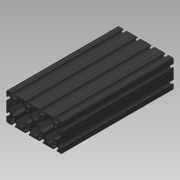
# Autodesk Inventor part: 3060
Saved by Autodesk Inventor 2013 (Build 170138000, 138)
## iProperties
Company: 80/20 Inc.
Created: 2014-04-23
Part Number: 3060
Material: Generic
Document SubType Name: Modeling
Density: 1 g/cm^3
Vendor: 80/20 Inc.
Engineer: Ross Bowman
Designer: Ross Bowman
Catalog Web Link: 8020.net
Material: 6105-T5 Aluminum
Author: Ross Bowman
Keywords: 80/20 , 8020 , T-Slot , Extrusion
Autodesk Inventor part; units mm, degrees
ref_plane "YZ Plane" through (0, 0, 0) normal (1, 0, 0) x (0, 1, 0)
ref_plane "XZ Plane" through (0, 0, 0) normal (0, 1, 0) x (-1, 0, 0)
ref_plane "XY Plane" through (0, 0, 0) normal (0, 0, 1) x (1, 0, 0)
sketch "Sketch1" plane through (0, 0, 0) normal (0, 0, 1) x (1, 0, 0)
  circle A0 centre (57.15, -19.05) radius 3.3274
  circle A1 centre (19.05, -19.05) radius 3.3274
  circle A2 centre (-57.15, 19.05) radius 3.3274
  circle A3 centre (-19.05, 19.05) radius 3.3274
  circle A4 centre (-19.05, -19.05) radius 3.3274
  circle A5 centre (-57.15, -19.05) radius 3.3274
  arc A6 (-51.5823, -18.8539) -> (-50.1854, -22.2287) centre (-46.8071, -18.8539) ccw
  line L0 (-51.5823, -15.4686) -> (-51.5823, -18.8539)
  arc A7 (-51.5823, -15.4686) -> (-54.7573, -12.2936) centre (-54.7573, -15.4686) ccw
  line L1 (-58.1099, -12.2936) -> (-54.7573, -12.2936)
  arc A8 (-61.4883, -10.8932) -> (-58.1099, -12.2936) centre (-58.1099, -7.5184) ccw
  line L2 (-70.3244, -2.0479) -> (-61.4883, -10.8932)
  arc A9 (-70.3244, 2.0479) -> (-70.3244, -2.0479) centre (-68.2744, 0) ccw
  line L3 (-61.4883, 10.8932) -> (-70.3244, 2.0479)
  arc A10 (-58.1099, 12.2936) -> (-61.4883, 10.8932) centre (-58.1099, 7.5184) ccw
  line L4 (-54.7573, 12.2936) -> (-58.1099, 12.2936)
  arc A11 (-54.7573, 12.2936) -> (-51.5823, 15.4686) centre (-54.7573, 15.4686) ccw
  line L5 (-51.5823, 18.8539) -> (-51.5823, 15.4686)
  arc A12 (-50.1854, 22.2287) -> (-51.5823, 18.8539) centre (-46.8071, 18.8539) ccw
  line L6 (-40.8869, 31.5369) -> (-50.1854, 22.2287)
  arc A13 (-36.3704, 31.5369) -> (-40.8869, 31.5369) centre (-38.6286, 29.281) ccw
  line L7 (-27.0718, 22.2287) -> (-36.3704, 31.5369)
  arc A14 (-25.675, 18.8539) -> (-27.0718, 22.2287) centre (-30.4502, 18.8539) ccw
  line L8 (-25.675, 15.4686) -> (-25.675, 18.8539)
  arc A15 (-25.675, 15.4686) -> (-22.5, 12.2936) centre (-22.5, 15.4686) ccw
  line L9 (-19.1368, 12.2936) -> (-22.5, 12.2936)
  arc A16 (-15.7765, 10.9007) -> (-19.1368, 12.2936) centre (-19.1368, 7.5438) ccw
  line L10 (-6.9329, 2.0479) -> (-15.7765, 10.9007)
  arc A17 (-6.9329, -2.0479) -> (-6.9329, 2.0479) centre (-8.9829, 0) ccw
  line L11 (-15.7765, -10.9007) -> (-6.9329, -2.0479)
  arc A18 (-19.1368, -12.2936) -> (-15.7765, -10.9007) centre (-19.1368, -7.5438) ccw
  line L12 (-22.5, -12.2936) -> (-19.1368, -12.2936)
  arc A19 (-22.5, -12.2936) -> (-25.675, -15.4686) centre (-22.5, -15.4686) ccw
  line L13 (-25.675, -18.8539) -> (-25.675, -15.4686)
  arc A20 (-27.0718, -22.2287) -> (-25.675, -18.8539) centre (-30.4502, -18.8539) ccw
  line L14 (-36.3704, -31.5369) -> (-27.0718, -22.2287)
  arc A21 (-40.8869, -31.5369) -> (-36.3704, -31.5369) centre (-38.6286, -29.281) ccw
  line L15 (-50.1854, -22.2287) -> (-40.8869, -31.5369)
  arc A22 (-3.7429, 5.5394) -> (3.7429, 5.5394) centre (0, 9.2784) ccw
  line L16 (-11.3507, 13.1551) -> (-3.7429, 5.5394)
  arc A23 (-12.425, 15.7507) -> (-11.3507, 13.1551) centre (-8.7523, 15.7507) ccw
  line L17 (-12.425, 22.3493) -> (-12.425, 15.7507)
  arc A24 (-11.3507, 24.9449) -> (-12.425, 22.3493) centre (-8.7523, 22.3493) ccw
  line L18 (-2.7156, 33.589) -> (-11.3507, 24.9449)
  arc A25 (2.7156, 33.589) -> (-2.7156, 33.589) centre (0, 30.8762) ccw
  line L19 (11.3507, 24.9449) -> (2.7156, 33.589)
  arc A26 (12.425, 22.3493) -> (11.3507, 24.9449) centre (8.7523, 22.3493) ccw
  line L20 (12.425, 15.7507) -> (12.425, 22.3493)
  arc A27 (11.3507, 13.1551) -> (12.425, 15.7507) centre (8.7523, 15.7507) ccw
  line L21 (3.7429, 5.5394) -> (11.3507, 13.1551)
  circle A28 centre (19.05, 19.05) radius 3.3274
  circle A29 centre (57.15, 19.05) radius 3.3274
  arc A30 (-2.7156, -33.589) -> (2.7156, -33.589) centre (0, -30.8762) ccw
  line L22 (-11.3507, -24.9449) -> (-2.7156, -33.589)
  arc A31 (-12.425, -22.3493) -> (-11.3507, -24.9449) centre (-8.7523, -22.3493) ccw
  line L23 (-12.425, -15.7507) -> (-12.425, -22.3493)
  arc A32 (-11.3507, -13.1551) -> (-12.425, -15.7507) centre (-8.7523, -15.7507) ccw
  line L24 (-3.7429, -5.5394) -> (-11.3507, -13.1551)
  arc A33 (3.7429, -5.5394) -> (-3.7429, -5.5394) centre (0, -9.2784) ccw
  line L25 (11.3507, -13.1551) -> (3.7429, -5.5394)
  arc A34 (12.425, -15.7507) -> (11.3507, -13.1551) centre (8.7523, -15.7507) ccw
  line L26 (12.425, -22.3493) -> (12.425, -15.7507)
  arc A35 (11.3507, -24.9449) -> (12.425, -22.3493) centre (8.7523, -22.3493) ccw
  line L27 (2.7156, -33.589) -> (11.3507, -24.9449)
  arc A36 (6.9329, 2.0479) -> (6.9329, -2.0479) centre (8.9829, 0) ccw
  line L28 (15.7765, 10.9007) -> (6.9329, 2.0479)
  arc A37 (19.1368, 12.2936) -> (15.7765, 10.9007) centre (19.1368, 7.5438) ccw
  line L29 (22.5, 12.2936) -> (19.1368, 12.2936)
  arc A38 (22.5, 12.2936) -> (25.675, 15.4686) centre (22.5, 15.4686) ccw
  line L30 (25.675, 18.8539) -> (25.675, 15.4686)
  arc A39 (27.0718, 22.2287) -> (25.675, 18.8539) centre (30.4502, 18.8539) ccw
  line L31 (36.3704, 31.5369) -> (27.0718, 22.2287)
  arc A40 (40.8869, 31.5369) -> (36.3704, 31.5369) centre (38.6286, 29.281) ccw
  line L32 (50.1854, 22.2287) -> (40.8869, 31.5369)
  arc A41 (51.5823, 18.8539) -> (50.1854, 22.2287) centre (46.8071, 18.8539) ccw
  line L33 (51.5823, 15.4686) -> (51.5823, 18.8539)
  arc A42 (51.5823, 15.4686) -> (54.7573, 12.2936) centre (54.7573, 15.4686) ccw
  line L34 (58.1099, 12.2936) -> (54.7573, 12.2936)
  arc A43 (61.4883, 10.8932) -> (58.1099, 12.2936) centre (58.1099, 7.5184) ccw
  line L35 (70.3244, 2.0479) -> (61.4883, 10.8932)
  arc A44 (70.3244, -2.0479) -> (70.3244, 2.0479) centre (68.2744, 0) ccw
  line L36 (61.4883, -10.8932) -> (70.3244, -2.0479)
  arc A45 (58.1099, -12.2936) -> (61.4883, -10.8932) centre (58.1099, -7.5184) ccw
  line L37 (54.7573, -12.2936) -> (58.1099, -12.2936)
  arc A46 (54.7573, -12.2936) -> (51.5823, -15.4686) centre (54.7573, -15.4686) ccw
  line L38 (51.5823, -18.8539) -> (51.5823, -15.4686)
  arc A47 (50.1854, -22.2287) -> (51.5823, -18.8539) centre (46.8071, -18.8539) ccw
  line L39 (40.8869, -31.5369) -> (50.1854, -22.2287)
  arc A48 (36.3704, -31.5369) -> (40.8869, -31.5369) centre (38.6286, -29.281) ccw
  line L40 (27.0718, -22.2287) -> (36.3704, -31.5369)
  arc A49 (25.675, -18.8539) -> (27.0718, -22.2287) centre (30.4502, -18.8539) ccw
  line L41 (25.675, -15.4686) -> (25.675, -18.8539)
  arc A50 (25.675, -15.4686) -> (22.5, -12.2936) centre (22.5, -15.4686) ccw
  line L42 (19.1368, -12.2936) -> (22.5, -12.2936)
  arc A51 (15.7765, -10.9007) -> (19.1368, -12.2936) centre (19.1368, -7.5438) ccw
  line L43 (6.9329, -2.0479) -> (15.7765, -10.9007)
  arc A52 (28.5292, -38.1) -> (27.0066, -38.1) centre (27.7679, -38.1) ccw
  line L44 (28.5292, -38.1) -> (33.4119, -38.1)
  arc A53 (34.9345, -38.1) -> (33.4119, -38.1) centre (34.1732, -38.1) ccw
  line L45 (34.9345, -38.1) -> (42.3228, -38.1)
  arc A54 (43.8453, -38.1) -> (42.3228, -38.1) centre (43.0841, -38.1) ccw
  line L46 (43.8453, -38.1) -> (47.5811, -38.1)
  arc A55 (49.1036, -38.1) -> (47.5811, -38.1) centre (48.3424, -38.1) ccw
  line L47 (49.1036, -38.1) -> (51.5112, -38.1)
  arc A56 (51.5112, -38.1) -> (53.086, -36.5252) centre (51.5112, -36.5252) ccw
  line L48 (53.086, -36.5252) -> (53.086, -35.6108)
  arc A57 (53.086, -35.6108) -> (51.5112, -34.036) centre (51.5112, -35.6108) ccw
  line L49 (51.5112, -34.036) -> (47.752, -34.036)
  arc A58 (46.863, -33.147) -> (47.752, -34.036) centre (47.752, -33.147) ccw
  line L50 (46.863, -33.147) -> (46.863, -32.5952)
  arc A59 (47.1231, -31.967) -> (46.863, -32.5952) centre (47.752, -32.5952) ccw
  line L51 (47.1231, -31.967) -> (51.9086, -27.1764)
  arc A60 (55.2137, -25.8064) -> (51.9086, -27.1764) centre (55.2137, -30.4782) ccw
  line L52 (55.2137, -25.8064) -> (59.0863, -25.8064)
  arc A61 (62.3914, -27.1764) -> (59.0863, -25.8064) centre (59.0863, -30.4782) ccw
  line L53 (62.3914, -27.1764) -> (67.1769, -31.967)
  arc A62 (67.437, -32.5952) -> (67.1769, -31.967) centre (66.548, -32.5952) ccw
  line L54 (67.437, -32.5952) -> (67.437, -33.147)
  arc A63 (66.548, -34.036) -> (67.437, -33.147) centre (66.548, -33.147) ccw
  line L55 (66.548, -34.036) -> (62.7888, -34.036)
  arc A64 (62.7888, -34.036) -> (61.214, -35.6108) centre (62.7888, -35.6108) ccw
  line L56 (61.214, -35.6108) -> (61.214, -36.5252)
  arc A65 (61.214, -36.5252) -> (62.7888, -38.1) centre (62.7888, -36.5252) ccw
  line L57 (62.7888, -38.1) -> (65.1067, -38.1)
  arc A66 (66.6292, -38.1) -> (65.1067, -38.1) centre (65.8679, -38.1) ccw
  line L58 (66.6292, -38.1) -> (71.4582, -38.1)
  arc A67 (72.9807, -38.1) -> (71.4582, -38.1) centre (72.2194, -38.1) ccw
  arc A68 (72.9807, -38.1) -> (76.2, -35.4576) centre (73.0698, -34.9262) ccw
  arc A69 (76.2, -33.935) -> (76.2, -35.4576) centre (76.2, -34.6963) ccw
  line L59 (76.2, -33.935) -> (76.2, -29.2617)
  arc A70 (76.2, -27.7391) -> (76.2, -29.2617) centre (76.2, -28.5004) ccw
  line L60 (76.2, -27.7391) -> (76.2, -24.6888)
  arc A71 (76.2, -24.6888) -> (74.6252, -23.114) centre (74.6252, -24.6888) ccw
  line L61 (74.6252, -23.114) -> (73.7108, -23.114)
  arc A72 (73.7108, -23.114) -> (72.136, -24.6888) centre (73.7108, -24.6888) ccw
  line L62 (72.136, -24.6888) -> (72.136, -29.1294)
  arc A73 (71.3385, -29.9269) -> (72.136, -29.1294) centre (71.3385, -29.1294) ccw
  line L63 (71.3385, -29.9269) -> (71.2424, -29.9269)
  arc A74 (70.6234, -29.6666) -> (71.2424, -29.9269) centre (71.2424, -29.0607) ccw
  line L64 (70.6234, -29.6666) -> (64.1071, -23.1436)
  arc A75 (62.7177, -19.7867) -> (64.1071, -23.1436) centre (67.4675, -19.7867) ccw
  line L65 (62.7177, -19.7867) -> (62.7177, -18.3133)
  arc A76 (64.1071, -14.9564) -> (62.7177, -18.3133) centre (67.4675, -18.3133) ccw
  line L66 (64.1071, -14.9564) -> (70.6297, -8.4271)
  arc A77 (71.2424, -8.1731) -> (70.6297, -8.4271) centre (71.2424, -9.0392) ccw
  line L67 (71.2424, -8.1731) -> (71.3385, -8.1731)
  arc A78 (72.136, -8.9706) -> (71.3385, -8.1731) centre (71.3385, -8.9706) ccw
  line L68 (72.136, -8.9706) -> (72.136, -13.4112)
  arc A79 (72.136, -13.4112) -> (73.7108, -14.986) centre (73.7108, -13.4112) ccw
  line L69 (73.7108, -14.986) -> (74.6252, -14.986)
  arc A80 (74.6252, -14.986) -> (76.2, -13.4112) centre (74.6252, -13.4112) ccw
  line L70 (76.2, -13.4112) -> (76.2, -11.7903)
  arc A81 (76.2, -10.2663) -> (76.2, -11.7903) centre (76.2, -11.0283) ccw
  line L71 (76.2, -10.2663) -> (76.2, -5.4385)
  arc A82 (76.2, -3.9149) -> (76.2, -5.4385) centre (76.2, -4.6767) ccw
  line L72 (76.2, -3.9149) -> (76.2, 3.9149)
  arc A83 (76.2, 5.4385) -> (76.2, 3.9149) centre (76.2, 4.6767) ccw
  line L73 (76.2, 5.4385) -> (76.2, 10.2663)
  arc A84 (76.2, 11.7903) -> (76.2, 10.2663) centre (76.2, 11.0283) ccw
  line L74 (76.2, 11.7903) -> (76.2, 13.4112)
  arc A85 (76.2, 13.4112) -> (74.6252, 14.986) centre (74.6252, 13.4112) ccw
  line L75 (74.6252, 14.986) -> (73.7108, 14.986)
  arc A86 (73.7108, 14.986) -> (72.136, 13.4112) centre (73.7108, 13.4112) ccw
  line L76 (72.136, 13.4112) -> (72.136, 8.9706)
  arc A87 (71.3385, 8.1731) -> (72.136, 8.9706) centre (71.3385, 8.9706) ccw
  line L77 (71.3385, 8.1731) -> (71.2424, 8.1731)
  arc A88 (70.6297, 8.4271) -> (71.2424, 8.1731) centre (71.2424, 9.0392) ccw
  line L78 (70.6297, 8.4271) -> (64.1071, 14.9564)
  arc A89 (62.7177, 18.3133) -> (64.1071, 14.9564) centre (67.4675, 18.3133) ccw
  line L79 (62.7177, 18.3133) -> (62.7177, 19.7867)
  arc A90 (64.1071, 23.1436) -> (62.7177, 19.7867) centre (67.4675, 19.7867) ccw
  line L80 (64.1071, 23.1436) -> (70.6234, 29.6666)
  arc A91 (71.2424, 29.9269) -> (70.6234, 29.6666) centre (71.2424, 29.0607) ccw
  line L81 (71.2424, 29.9269) -> (71.3385, 29.9269)
  arc A92 (72.136, 29.1294) -> (71.3385, 29.9269) centre (71.3385, 29.1294) ccw
  line L82 (72.136, 29.1294) -> (72.136, 24.6888)
  arc A93 (72.136, 24.6888) -> (73.7108, 23.114) centre (73.7108, 24.6888) ccw
  line L83 (73.7108, 23.114) -> (74.6252, 23.114)
  arc A94 (74.6252, 23.114) -> (76.2, 24.6888) centre (74.6252, 24.6888) ccw
  line L84 (76.2, 24.6888) -> (76.2, 27.7391)
  arc A95 (76.2, 29.2617) -> (76.2, 27.7391) centre (76.2, 28.5004) ccw
  line L85 (76.2, 29.2617) -> (76.2, 33.935)
  arc A96 (76.2, 35.4576) -> (76.2, 33.935) centre (76.2, 34.6963) ccw
  arc A97 (76.2, 35.4576) -> (72.9807, 38.1) centre (73.0698, 34.9262) ccw
  arc A98 (71.4582, 38.1) -> (72.9807, 38.1) centre (72.2194, 38.1) ccw
  line L86 (71.4582, 38.1) -> (66.6292, 38.1)
  arc A99 (65.1067, 38.1) -> (66.6292, 38.1) centre (65.8679, 38.1) ccw
  line L87 (65.1067, 38.1) -> (62.7888, 38.1)
  arc A100 (62.7888, 38.1) -> (61.214, 36.5252) centre (62.7888, 36.5252) ccw
  line L88 (61.214, 36.5252) -> (61.214, 35.6108)
  arc A101 (61.214, 35.6108) -> (62.7888, 34.036) centre (62.7888, 35.6108) ccw
  line L89 (62.7888, 34.036) -> (66.548, 34.036)
  arc A102 (67.437, 33.147) -> (66.548, 34.036) centre (66.548, 33.147) ccw
  line L90 (67.437, 33.147) -> (67.437, 32.5952)
  arc A103 (67.1769, 31.967) -> (67.437, 32.5952) centre (66.548, 32.5952) ccw
  line L91 (67.1769, 31.967) -> (62.3914, 27.1764)
  arc A104 (59.0863, 25.8064) -> (62.3914, 27.1764) centre (59.0863, 30.4782) ccw
  line L92 (59.0863, 25.8064) -> (55.2137, 25.8064)
  arc A105 (51.9086, 27.1764) -> (55.2137, 25.8064) centre (55.2137, 30.4782) ccw
  line L93 (51.9086, 27.1764) -> (47.1231, 31.967)
  arc A106 (46.863, 32.5952) -> (47.1231, 31.967) centre (47.752, 32.5952) ccw
  line L94 (46.863, 32.5952) -> (46.863, 33.147)
  arc A107 (47.752, 34.036) -> (46.863, 33.147) centre (47.752, 33.147) ccw
  line L95 (47.752, 34.036) -> (51.5112, 34.036)
  arc A108 (51.5112, 34.036) -> (53.086, 35.6108) centre (51.5112, 35.6108) ccw
  line L96 (53.086, 35.6108) -> (53.086, 36.5252)
  arc A109 (53.086, 36.5252) -> (51.5112, 38.1) centre (51.5112, 36.5252) ccw
  line L97 (51.5112, 38.1) -> (49.1036, 38.1)
  arc A110 (47.5811, 38.1) -> (49.1036, 38.1) centre (48.3424, 38.1) ccw
  line L98 (47.5811, 38.1) -> (43.8453, 38.1)
  arc A111 (42.3228, 38.1) -> (43.8453, 38.1) centre (43.0841, 38.1) ccw
  line L99 (42.3228, 38.1) -> (34.9345, 38.1)
  arc A112 (33.4119, 38.1) -> (34.9345, 38.1) centre (34.1732, 38.1) ccw
  line L100 (33.4119, 38.1) -> (28.5292, 38.1)
  arc A113 (27.0066, 38.1) -> (28.5292, 38.1) centre (27.7679, 38.1) ccw
  line L101 (27.0066, 38.1) -> (24.6888, 38.1)
  arc A114 (24.6888, 38.1) -> (23.114, 36.5252) centre (24.6888, 36.5252) ccw
  line L102 (23.114, 36.5252) -> (23.114, 35.6108)
  arc A115 (23.114, 35.6108) -> (24.6888, 34.036) centre (24.6888, 35.6108) ccw
  line L103 (24.6888, 34.036) -> (28.448, 34.036)
  arc A116 (29.337, 33.147) -> (28.448, 34.036) centre (28.448, 33.147) ccw
  line L104 (29.337, 33.147) -> (29.337, 32.9805)
  arc A117 (29.0769, 32.3522) -> (29.337, 32.9805) centre (28.448, 32.9805) ccw
  line L105 (29.0769, 32.3522) -> (23.9294, 27.1993)
  arc A118 (20.5691, 25.8064) -> (23.9294, 27.1993) centre (20.5691, 30.5562) ccw
  line L106 (20.5691, 25.8064) -> (17.5309, 25.8064)
  arc A119 (14.1706, 27.1993) -> (17.5309, 25.8064) centre (17.5309, 30.5562) ccw
  line L107 (14.1706, 27.1993) -> (9.0231, 32.3522)
  arc A120 (8.763, 32.9805) -> (9.0231, 32.3522) centre (9.652, 32.9805) ccw
  line L108 (8.763, 32.9805) -> (8.763, 33.147)
  arc A121 (9.652, 34.036) -> (8.763, 33.147) centre (9.652, 33.147) ccw
  line L109 (9.652, 34.036) -> (13.4112, 34.036)
  arc A122 (13.4112, 34.036) -> (14.986, 35.6108) centre (13.4112, 35.6108) ccw
  line L110 (14.986, 35.6108) -> (14.986, 36.4702)
  arc A123 (14.986, 36.4702) -> (13.4122, 38.1) centre (13.4122, 36.5252) ccw
  line L111 (13.4122, 38.1) -> (11.0569, 38.1)
  arc A124 (9.5343, 38.1) -> (11.0569, 38.1) centre (10.2956, 38.1) ccw
  line L112 (9.5343, 38.1) -> (4.6578, 38.1)
  arc A125 (3.1353, 38.1) -> (4.6578, 38.1) centre (3.8965, 38.1) ccw
  line L113 (3.1353, 38.1) -> (-3.1353, 38.1)
  arc A126 (-4.6578, 38.1) -> (-3.1353, 38.1) centre (-3.8965, 38.1) ccw
  line L114 (-4.6578, 38.1) -> (-9.5343, 38.1)
  arc A127 (-11.0569, 38.1) -> (-9.5343, 38.1) centre (-10.2956, 38.1) ccw
  line L115 (-11.0569, 38.1) -> (-13.4122, 38.1)
  arc A128 (-13.4122, 38.1) -> (-14.986, 36.4702) centre (-13.4122, 36.5252) ccw
  line L116 (-14.986, 36.4702) -> (-14.986, 35.6108)
  arc A129 (-14.986, 35.6108) -> (-13.4112, 34.036) centre (-13.4112, 35.6108) ccw
  line L117 (-13.4112, 34.036) -> (-9.652, 34.036)
  arc A130 (-8.763, 33.147) -> (-9.652, 34.036) centre (-9.652, 33.147) ccw
  line L118 (-8.763, 33.147) -> (-8.763, 32.9805)
  arc A131 (-9.0231, 32.3522) -> (-8.763, 32.9805) centre (-9.652, 32.9805) ccw
  line L119 (-9.0231, 32.3522) -> (-14.1706, 27.1993)
  arc A132 (-17.5309, 25.8064) -> (-14.1706, 27.1993) centre (-17.5309, 30.5562) ccw
  line L120 (-17.5309, 25.8064) -> (-20.5691, 25.8064)
  arc A133 (-23.9294, 27.1993) -> (-20.5691, 25.8064) centre (-20.5691, 30.5562) ccw
  line L121 (-23.9294, 27.1993) -> (-29.0769, 32.3522)
  arc A134 (-29.337, 32.9805) -> (-29.0769, 32.3522) centre (-28.448, 32.9805) ccw
  line L122 (-29.337, 32.9805) -> (-29.337, 33.147)
  arc A135 (-28.448, 34.036) -> (-29.337, 33.147) centre (-28.448, 33.147) ccw
  line L123 (-28.448, 34.036) -> (-24.6888, 34.036)
  arc A136 (-24.6888, 34.036) -> (-23.114, 35.6108) centre (-24.6888, 35.6108) ccw
  line L124 (-23.114, 35.6108) -> (-23.114, 36.5252)
  arc A137 (-23.114, 36.5252) -> (-24.6888, 38.1) centre (-24.6888, 36.5252) ccw
  line L125 (-24.6888, 38.1) -> (-27.0066, 38.1)
  arc A138 (-28.5292, 38.1) -> (-27.0066, 38.1) centre (-27.7679, 38.1) ccw
  line L126 (-28.5292, 38.1) -> (-33.4119, 38.1)
  arc A139 (-34.9345, 38.1) -> (-33.4119, 38.1) centre (-34.1732, 38.1) ccw
  line L127 (-34.9345, 38.1) -> (-42.3228, 38.1)
  arc A140 (-43.8453, 38.1) -> (-42.3228, 38.1) centre (-43.0841, 38.1) ccw
  line L128 (-43.8453, 38.1) -> (-47.5811, 38.1)
  arc A141 (-49.1036, 38.1) -> (-47.5811, 38.1) centre (-48.3424, 38.1) ccw
  line L129 (-49.1036, 38.1) -> (-51.5112, 38.1)
  arc A142 (-51.5112, 38.1) -> (-53.086, 36.5252) centre (-51.5112, 36.5252) ccw
  line L130 (-53.086, 36.5252) -> (-53.086, 35.6108)
  arc A143 (-53.086, 35.6108) -> (-51.5112, 34.036) centre (-51.5112, 35.6108) ccw
  line L131 (-51.5112, 34.036) -> (-47.752, 34.036)
  arc A144 (-46.863, 33.147) -> (-47.752, 34.036) centre (-47.752, 33.147) ccw
  line L132 (-46.863, 33.147) -> (-46.863, 32.5952)
  arc A145 (-47.1231, 31.967) -> (-46.863, 32.5952) centre (-47.752, 32.5952) ccw
  line L133 (-47.1231, 31.967) -> (-51.9086, 27.1764)
  arc A146 (-55.2137, 25.8064) -> (-51.9086, 27.1764) centre (-55.2137, 30.4782) ccw
  line L134 (-55.2137, 25.8064) -> (-59.0863, 25.8064)
  arc A147 (-62.3914, 27.1764) -> (-59.0863, 25.8064) centre (-59.0863, 30.4782) ccw
  line L135 (-62.3914, 27.1764) -> (-67.1769, 31.967)
  arc A148 (-67.437, 32.5952) -> (-67.1769, 31.967) centre (-66.548, 32.5952) ccw
  line L136 (-67.437, 32.5952) -> (-67.437, 33.147)
  arc A149 (-66.548, 34.036) -> (-67.437, 33.147) centre (-66.548, 33.147) ccw
  line L137 (-66.548, 34.036) -> (-62.7888, 34.036)
  arc A150 (-62.7888, 34.036) -> (-61.214, 35.6108) centre (-62.7888, 35.6108) ccw
  line L138 (-61.214, 35.6108) -> (-61.214, 36.5252)
  arc A151 (-61.214, 36.5252) -> (-62.7888, 38.1) centre (-62.7888, 36.5252) ccw
  line L139 (-62.7888, 38.1) -> (-65.1067, 38.1)
  arc A152 (-66.6292, 38.1) -> (-65.1067, 38.1) centre (-65.8679, 38.1) ccw
  line L140 (-66.6292, 38.1) -> (-71.4582, 38.1)
  arc A153 (-72.9807, 38.1) -> (-71.4582, 38.1) centre (-72.2194, 38.1) ccw
  arc A154 (-72.9807, 38.1) -> (-76.2, 35.4576) centre (-73.0698, 34.9262) ccw
  arc A155 (-76.2, 33.935) -> (-76.2, 35.4576) centre (-76.2, 34.6963) ccw
  line L141 (-76.2, 33.935) -> (-76.2, 29.2617)
  arc A156 (-76.2, 27.7391) -> (-76.2, 29.2617) centre (-76.2, 28.5004) ccw
  line L142 (-76.2, 27.7391) -> (-76.2, 24.6888)
  arc A157 (-76.2, 24.6888) -> (-74.6252, 23.114) centre (-74.6252, 24.6888) ccw
  line L143 (-74.6252, 23.114) -> (-73.7108, 23.114)
  arc A158 (-73.7108, 23.114) -> (-72.136, 24.6888) centre (-73.7108, 24.6888) ccw
  line L144 (-72.136, 24.6888) -> (-72.136, 29.1294)
  arc A159 (-71.3385, 29.9269) -> (-72.136, 29.1294) centre (-71.3385, 29.1294) ccw
  line L145 (-71.3385, 29.9269) -> (-71.2424, 29.9269)
  arc A160 (-70.6234, 29.6666) -> (-71.2424, 29.9269) centre (-71.2424, 29.0607) ccw
  line L146 (-70.6234, 29.6666) -> (-64.1071, 23.1436)
  arc A161 (-62.7177, 19.7867) -> (-64.1071, 23.1436) centre (-67.4675, 19.7867) ccw
  line L147 (-62.7177, 19.7867) -> (-62.7177, 18.3133)
  arc A162 (-64.1071, 14.9564) -> (-62.7177, 18.3133) centre (-67.4675, 18.3133) ccw
  line L148 (-64.1071, 14.9564) -> (-70.6297, 8.4271)
  arc A163 (-71.2424, 8.1731) -> (-70.6297, 8.4271) centre (-71.2424, 9.0392) ccw
  line L149 (-71.2424, 8.1731) -> (-71.3385, 8.1731)
  arc A164 (-72.136, 8.9706) -> (-71.3385, 8.1731) centre (-71.3385, 8.9706) ccw
  line L150 (-72.136, 8.9706) -> (-72.136, 13.4112)
  arc A165 (-72.136, 13.4112) -> (-73.7108, 14.986) centre (-73.7108, 13.4112) ccw
  line L151 (-73.7108, 14.986) -> (-74.6252, 14.986)
  arc A166 (-74.6252, 14.986) -> (-76.2, 13.4112) centre (-74.6252, 13.4112) ccw
  line L152 (-76.2, 13.4112) -> (-76.2, 11.7903)
  arc A167 (-76.2, 10.2663) -> (-76.2, 11.7903) centre (-76.2, 11.0283) ccw
  line L153 (-76.2, 10.2663) -> (-76.2, 5.4385)
  arc A168 (-76.2, 3.9149) -> (-76.2, 5.4385) centre (-76.2, 4.6767) ccw
  line L154 (-76.2, 3.9149) -> (-76.2, -3.9149)
  arc A169 (-76.2, -5.4385) -> (-76.2, -3.9149) centre (-76.2, -4.6767) ccw
  line L155 (-76.2, -5.4385) -> (-76.2, -10.2663)
  arc A170 (-76.2, -11.7903) -> (-76.2, -10.2663) centre (-76.2, -11.0283) ccw
  line L156 (-76.2, -11.7903) -> (-76.2, -13.4112)
  arc A171 (-76.2, -13.4112) -> (-74.6252, -14.986) centre (-74.6252, -13.4112) ccw
  line L157 (-74.6252, -14.986) -> (-73.7108, -14.986)
  arc A172 (-73.7108, -14.986) -> (-72.136, -13.4112) centre (-73.7108, -13.4112) ccw
  line L158 (-72.136, -13.4112) -> (-72.136, -8.9706)
  arc A173 (-71.3385, -8.1731) -> (-72.136, -8.9706) centre (-71.3385, -8.9706) ccw
  line L159 (-71.3385, -8.1731) -> (-71.2424, -8.1731)
  arc A174 (-70.6297, -8.4271) -> (-71.2424, -8.1731) centre (-71.2424, -9.0392) ccw
  line L160 (-70.6297, -8.4271) -> (-64.1071, -14.9564)
  arc A175 (-62.7177, -18.3133) -> (-64.1071, -14.9564) centre (-67.4675, -18.3133) ccw
  line L161 (-62.7177, -18.3133) -> (-62.7177, -19.7867)
  arc A176 (-64.1071, -23.1436) -> (-62.7177, -19.7867) centre (-67.4675, -19.7867) ccw
  line L162 (-64.1071, -23.1436) -> (-70.6234, -29.6666)
  arc A177 (-71.2424, -29.9269) -> (-70.6234, -29.6666) centre (-71.2424, -29.0607) ccw
  line L163 (-71.2424, -29.9269) -> (-71.3385, -29.9269)
  arc A178 (-72.136, -29.1294) -> (-71.3385, -29.9269) centre (-71.3385, -29.1294) ccw
  line L164 (-72.136, -29.1294) -> (-72.136, -24.6888)
  arc A179 (-72.136, -24.6888) -> (-73.7108, -23.114) centre (-73.7108, -24.6888) ccw
  line L165 (-73.7108, -23.114) -> (-74.6252, -23.114)
  arc A180 (-74.6252, -23.114) -> (-76.2, -24.6888) centre (-74.6252, -24.6888) ccw
  line L166 (-76.2, -24.6888) -> (-76.2, -27.7391)
  arc A181 (-76.2, -29.2617) -> (-76.2, -27.7391) centre (-76.2, -28.5004) ccw
  line L167 (-76.2, -29.2617) -> (-76.2, -33.935)
  arc A182 (-76.2, -35.4576) -> (-76.2, -33.935) centre (-76.2, -34.6963) ccw
  arc A183 (-76.2, -35.4576) -> (-72.9807, -38.1) centre (-73.0698, -34.9262) ccw
  arc A184 (-71.4582, -38.1) -> (-72.9807, -38.1) centre (-72.2194, -38.1) ccw
  line L168 (-71.4582, -38.1) -> (-66.6292, -38.1)
  arc A185 (-65.1067, -38.1) -> (-66.6292, -38.1) centre (-65.8679, -38.1) ccw
  line L169 (-65.1067, -38.1) -> (-62.7888, -38.1)
  arc A186 (-62.7888, -38.1) -> (-61.214, -36.5252) centre (-62.7888, -36.5252) ccw
  line L170 (-61.214, -36.5252) -> (-61.214, -35.6108)
  arc A187 (-61.214, -35.6108) -> (-62.7888, -34.036) centre (-62.7888, -35.6108) ccw
  line L171 (-62.7888, -34.036) -> (-66.548, -34.036)
  arc A188 (-67.437, -33.147) -> (-66.548, -34.036) centre (-66.548, -33.147) ccw
  line L172 (-67.437, -33.147) -> (-67.437, -32.5952)
  arc A189 (-67.1769, -31.967) -> (-67.437, -32.5952) centre (-66.548, -32.5952) ccw
  line L173 (-67.1769, -31.967) -> (-62.3914, -27.1764)
  arc A190 (-59.0863, -25.8064) -> (-62.3914, -27.1764) centre (-59.0863, -30.4782) ccw
  line L174 (-59.0863, -25.8064) -> (-55.2137, -25.8064)
  arc A191 (-51.9086, -27.1764) -> (-55.2137, -25.8064) centre (-55.2137, -30.4782) ccw
  line L175 (-51.9086, -27.1764) -> (-47.1231, -31.967)
  arc A192 (-46.863, -32.5952) -> (-47.1231, -31.967) centre (-47.752, -32.5952) ccw
  line L176 (-46.863, -32.5952) -> (-46.863, -33.147)
  arc A193 (-47.752, -34.036) -> (-46.863, -33.147) centre (-47.752, -33.147) ccw
  line L177 (-47.752, -34.036) -> (-51.5112, -34.036)
  arc A194 (-51.5112, -34.036) -> (-53.086, -35.6108) centre (-51.5112, -35.6108) ccw
  line L178 (-53.086, -35.6108) -> (-53.086, -36.5252)
  arc A195 (-53.086, -36.5252) -> (-51.5112, -38.1) centre (-51.5112, -36.5252) ccw
  line L179 (-51.5112, -38.1) -> (-49.1036, -38.1)
  arc A196 (-47.5811, -38.1) -> (-49.1036, -38.1) centre (-48.3424, -38.1) ccw
  line L180 (-47.5811, -38.1) -> (-43.8453, -38.1)
  arc A197 (-42.3228, -38.1) -> (-43.8453, -38.1) centre (-43.0841, -38.1) ccw
  line L181 (-42.3228, -38.1) -> (-34.9345, -38.1)
  arc A198 (-33.4119, -38.1) -> (-34.9345, -38.1) centre (-34.1732, -38.1) ccw
  line L182 (-33.4119, -38.1) -> (-28.5292, -38.1)
  arc A199 (-27.0066, -38.1) -> (-28.5292, -38.1) centre (-27.7679, -38.1) ccw
  line L183 (-27.0066, -38.1) -> (-24.6888, -38.1)
  arc A200 (-24.6888, -38.1) -> (-23.114, -36.5252) centre (-24.6888, -36.5252) ccw
  line L184 (-23.114, -36.5252) -> (-23.114, -35.6108)
  arc A201 (-23.114, -35.6108) -> (-24.6888, -34.036) centre (-24.6888, -35.6108) ccw
  line L185 (-24.6888, -34.036) -> (-28.448, -34.036)
  arc A202 (-29.337, -33.147) -> (-28.448, -34.036) centre (-28.448, -33.147) ccw
  line L186 (-29.337, -33.147) -> (-29.337, -32.9805)
  arc A203 (-29.0769, -32.3522) -> (-29.337, -32.9805) centre (-28.448, -32.9805) ccw
  line L187 (-29.0769, -32.3522) -> (-23.9294, -27.1993)
  arc A204 (-20.5691, -25.8064) -> (-23.9294, -27.1993) centre (-20.5691, -30.5562) ccw
  line L188 (-20.5691, -25.8064) -> (-17.5309, -25.8064)
  arc A205 (-14.1706, -27.1993) -> (-17.5309, -25.8064) centre (-17.5309, -30.5562) ccw
  line L189 (-14.1706, -27.1993) -> (-9.0231, -32.3522)
  arc A206 (-8.763, -32.9805) -> (-9.0231, -32.3522) centre (-9.652, -32.9805) ccw
  line L190 (-8.763, -32.9805) -> (-8.763, -33.147)
  arc A207 (-9.652, -34.036) -> (-8.763, -33.147) centre (-9.652, -33.147) ccw
  line L191 (-9.652, -34.036) -> (-13.4112, -34.036)
  arc A208 (-13.4112, -34.036) -> (-14.986, -35.6108) centre (-13.4112, -35.6108) ccw
  line L192 (-14.986, -35.6108) -> (-14.986, -36.4702)
  arc A209 (-14.986, -36.4702) -> (-13.4122, -38.1) centre (-13.4122, -36.5252) ccw
  line L193 (-13.4122, -38.1) -> (-11.0569, -38.1)
  arc A210 (-9.5343, -38.1) -> (-11.0569, -38.1) centre (-10.2956, -38.1) ccw
  line L194 (-9.5343, -38.1) -> (-4.6578, -38.1)
  arc A211 (-3.1353, -38.1) -> (-4.6578, -38.1) centre (-3.8965, -38.1) ccw
  line L195 (-3.1353, -38.1) -> (3.1353, -38.1)
  arc A212 (4.6578, -38.1) -> (3.1353, -38.1) centre (3.8965, -38.1) ccw
  line L196 (4.6578, -38.1) -> (9.5343, -38.1)
  arc A213 (11.0569, -38.1) -> (9.5343, -38.1) centre (10.2956, -38.1) ccw
  line L197 (11.0569, -38.1) -> (13.4122, -38.1)
  arc A214 (13.4122, -38.1) -> (14.986, -36.4702) centre (13.4122, -36.5252) ccw
  line L198 (14.986, -36.4702) -> (14.986, -35.6108)
  arc A215 (14.986, -35.6108) -> (13.4112, -34.036) centre (13.4112, -35.6108) ccw
  line L199 (13.4112, -34.036) -> (9.652, -34.036)
  arc A216 (8.763, -33.147) -> (9.652, -34.036) centre (9.652, -33.147) ccw
  line L200 (8.763, -33.147) -> (8.763, -32.9805)
  arc A217 (9.0231, -32.3522) -> (8.763, -32.9805) centre (9.652, -32.9805) ccw
  line L201 (9.0231, -32.3522) -> (14.1706, -27.1993)
  arc A218 (17.5309, -25.8064) -> (14.1706, -27.1993) centre (17.5309, -30.5562) ccw
  line L202 (17.5309, -25.8064) -> (20.5691, -25.8064)
  arc A219 (23.9294, -27.1993) -> (20.5691, -25.8064) centre (20.5691, -30.5562) ccw
  line L203 (23.9294, -27.1993) -> (29.0769, -32.3522)
  arc A220 (29.337, -32.9805) -> (29.0769, -32.3522) centre (28.448, -32.9805) ccw
  line L204 (29.337, -32.9805) -> (29.337, -33.147)
  arc A221 (28.448, -34.036) -> (29.337, -33.147) centre (28.448, -33.147) ccw
  line L205 (28.448, -34.036) -> (24.6888, -34.036)
  arc A222 (24.6888, -34.036) -> (23.114, -35.6108) centre (24.6888, -35.6108) ccw
  line L206 (23.114, -35.6108) -> (23.114, -36.5252)
  arc A223 (23.114, -36.5252) -> (24.6888, -38.1) centre (24.6888, -36.5252) ccw
  line L207 (24.6888, -38.1) -> (27.0066, -38.1)
  point P0 (0, 0)
  constraints: 432 point on circle, 416 end point, 224 centre point
extrude "Extrusion1" add sketch "Sketch1" against normal blind 304.8
body "Solid1"
